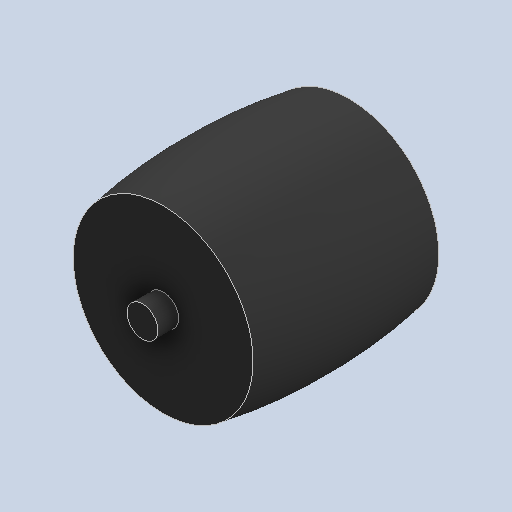
# Autodesk Inventor part: omuni_rubber
Saved by Autodesk Inventor 2025.1 (Build 291241000, 241)
## iProperties
Created: 2023-11-21
Part Number: omuni_rubber
Material: ゴム
Document SubType Name: Modeling
Designer: fhbdh
Density: 0.93 g/cm^3
Appearance: ゴム - 黒
Author: fhbdh
Autodesk Inventor part; units mm, degrees
ref_plane "YZ Plane" through (0, 0, 0) normal (1, 0, 0) x (0, 1, 0)
ref_plane "XZ Plane" through (0, 0, 0) normal (0, 1, 0) x (-1, 0, 0)
ref_plane "XY Plane" through (0, 0, 0) normal (0, 0, 1) x (1, 0, 0)
sketch "スケッチ1" plane through (0, 0, 0) normal (1, 0, 0) x (0, 1, 0)
  line L0 (-9.5, -9) -> (9.5, -9)
  line L1 (9.5, -9) -> (9.5, 9)
  line L2 (9.5, 9) -> (-9.5, 9)
  line L3 (-9.5, 9) -> (-9.5, -9)
  line L4 (-9.5, -9) -> (9.5, 9) construction
  line L5 (9.5, -9) -> (-9.5, 9) construction
  circle A0 centre (-43, 0) radius 52.5
  line L6 (0, 0) -> (-43, 0) construction
  circle A1 centre (43, 0) radius 52.5
  line L7 (0, 9) -> (0, -9)
  point P0 (9.5, 0)
  point P1 (-9.5, 0)
  point P2 (-8.7228, 9)
  point P3 (-8.7228, -9)
  dimension "d2" = 105
  dimension "d3" = 105
  dimension "d0" = 19
  dimension "d1" = 18
  constraints: 16 end point, 6 midpoint, 2 horizontal, 2 parallel, 1 horizontal alignment, 1 perpendicular, 1 point on line, 5 other
  measures "d0" distance of L1.end L2.end
  measures "d1" distance of L0.end L1.end
revolve "回転1" add sketch "スケッチ1" angle 360 about axis through (0, 0, 9) along (0, 0, -1) contours A1 L2 L7 L0
sketch "スケッチ2" plane through (0, 0, 9) normal (0, 0, 1) x (1, 0, 0)
  circle A0 centre (0, 0) radius 1.5
  dimension "d5" = 3
  constraints: 1 centre point, 1 coincident
  measures "d5" diameter of A0
sketch "スケッチ3" plane through (0, 0, -9) normal (0, 0, -1) x (-1, 0, 0)
  circle A0 centre (0, 0) radius 1.5
  dimension "d6" = 3
  constraints: 1 centre point, 1 coincident
  measures "d6" diameter of A0
extrude "押し出し1" add sketch "スケッチ2" along normal blind 2
extrude "押し出し2" add sketch "スケッチ3" along normal blind 2
equation "\"d3\" = d2"
